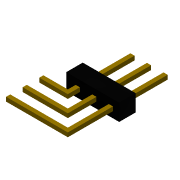
# Autodesk Inventor part: HeaderRight3
Saved by Autodesk Inventor 2015 (Build 190159000, 159)
## iProperties
Created: 2014-08-02
Part Number: HeaderRight3
Material: Generic
Document SubType Name: Modeling
Designer: david
Density: 1 g/cm^3
Appearance: Black
Author: david
Autodesk Inventor part; units mm, degrees
ref_plane "YZ Plane" through (0, 0, 0) normal (1, 0, 0) x (0, 1, 0)
ref_plane "XZ Plane" through (0, 0, 0) normal (0, 1, 0) x (-1, 0, 0)
ref_plane "XY Plane" through (0, 0, 0) normal (0, 0, 1) x (1, 0, 0)
sketch "Sketch1" plane through (0, 0, 0) normal (0, 1, 0) x (-1, 0, 0)
  line L0 (-1.4605, -5.842) -> (-2.0955, -5.842)
  line L1 (-2.0955, -5.842) -> (-2.0955, 4.3815)
  line L2 (-2.0955, 4.3815) -> (2.286, 4.3815)
  line L3 (2.286, 4.3815) -> (2.286, 3.7465)
  line L4 (2.286, 3.7465) -> (-1.4605, 3.7465)
  line L5 (-1.4605, 3.7465) -> (-1.4605, -5.842)
  line L6 (2.286, 6.2865) -> (2.286, 6.9215)
  line L7 (2.286, 6.9215) -> (-4.6355, 6.9215)
  line L8 (-4.6355, 6.9215) -> (-4.6355, -5.842)
  line L9 (-4.6355, -5.842) -> (-4.0005, -5.842)
  line L10 (-4.0005, -5.842) -> (-4.0005, 6.2865)
  line L11 (-4.0005, 6.2865) -> (2.286, 6.2865)
  line L12 (2.286, 8.8265) -> (2.286, 9.4615)
  line L13 (2.286, 9.4615) -> (-7.1755, 9.4615)
  line L14 (-7.1755, 9.4615) -> (-7.1755, -5.842)
  line L15 (-7.1755, -5.842) -> (-6.5405, -5.842)
  line L16 (-6.5405, -5.842) -> (-6.5405, 8.8265)
  line L17 (-6.5405, 8.8265) -> (2.286, 8.8265)
  line L18 (2.286, 4.064) -> (9.1077, 4.064) construction
  line L19 (2.286, 6.604) -> (8.649, 6.604) construction
  line L20 (2.286, 9.144) -> (8.4197, 9.144) construction
  line L21 (-1.778, -5.842) -> (-1.778, -10.327) construction
  line L22 (-4.318, -5.842) -> (-4.318, -10.188) construction
  line L23 (-6.858, -5.842) -> (-6.858, -10.8865) construction
  line L24 (12.5548, 0) -> (-11.5751, 0) construction
  line L25 (0, -14.9561) -> (0, 13.5311) construction
  line L26 (0, 0) -> (-8.128, 0) construction
  line L27 (-8.128, 0) -> (-8.128, 2.54) construction
  line L28 (-8.128, 2.54) -> (0, 2.54) construction
  line L29 (0, 2.54) -> (0, 0) construction
  line L30 (-2.54, 0) -> (-2.54, 2.54) construction
  dimension "d24" = 2.54
  dimension "d25" = 2.54
  dimension "d26" = 2.54
  dimension "d27" = 2.54
  dimension "d29" = 0.635
  dimension "d30" = 5.842
  dimension "d32" = 2.54
  dimension "d33" = 8.128
  dimension "d34" = 2.286
  dimension "d35" = 1.778
  dimension "d36" = 1.524
  dimension "d44" = 2.54
  dimension "d45" = 4.826
  constraints: 58 end point, 16 perpendicular, 6 midpoint, 5 equal length, 5 horizontal, 5 vertical, 4 collinear, 4 point on line, 3 parallel
  measures "d24" distance between parallel lines of L19 L18
  measures "d25" distance between parallel lines of L20 L19
  measures "d26" distance between parallel lines of L22 L21
  measures "d27" distance between parallel lines of L23 L22
  measures "d29" distance between parallel lines of L4 L2
  measures "d30" distance between parallel lines of L24 L0
  measures "d32" distance of L28.end L26.start
  measures "d33" distance of L26.start L26.end
  measures "d34" distance between parallel lines of L29 L3
  measures "d35" distance from line of L25 L21.start
  measures "d36" distance between parallel lines of L28 L18
  measures "d44" distance between parallel lines of L29 L30
  measures "d45" distance between parallel lines of L30 L6
extrude "Extrusion1" add sketch "Sketch1" along normal mid plane 0.635
sketch "Sketch3" plane through (0, 0, 0) normal (0, 0, 1) x (1, 0, 0)
  line L0 (0, -1.27) -> (8.128, -1.27)
  line L1 (8.128, -1.27) -> (8.128, 1.27)
  line L2 (8.128, 1.27) -> (0, 1.27)
  line L3 (0, 1.27) -> (0, -1.27)
  line L4 (1.4605, 0.3175) -> (1.4605, -0.3175) projected
  line L5 (1.4605, -0.3175) -> (1.4605, 0.3175) projected
  line L6 (2.0955, 0.3175) -> (1.4605, 0.3175) projected
  line L7 (1.4605, 0.3175) -> (-2.286, 0.3175) projected
  line L8 (-2.286, 0.3175) -> (2.0955, 0.3175) projected
  line L9 (1.4605, -0.3175) -> (2.0955, -0.3175) projected
  line L10 (2.0955, -0.3175) -> (-2.286, -0.3175) projected
  line L11 (-2.286, -0.3175) -> (1.4605, -0.3175) projected
  line L12 (1.4605, 0) -> (0, 0) construction
  line L13 (7.1755, -0.3175) -> (7.1755, 0.3175) construction
  line L14 (7.1755, -0.3175) -> (7.1755, 0.3175) construction
  point P0 (0, 0)
  dimension "d37" = 2.54
  dimension "d38" = 8.128
  dimension "d39" = 1.4605
  dimension "d40" = 0.9525
  constraints: 10 end point, 2 horizontal, 2 midpoint, 2 parallel, 1 perpendicular
  measures "d37" distance of L0.end L1.end
  measures "d38" distance of L1.end L2.end
  measures "d39" distance between parallel lines of L5 L3
  measures "d40" distance between parallel lines of L1 L13
extrude "Extrusion3" add sketch "Sketch3" along normal blind 2.54
body "Solid1"
